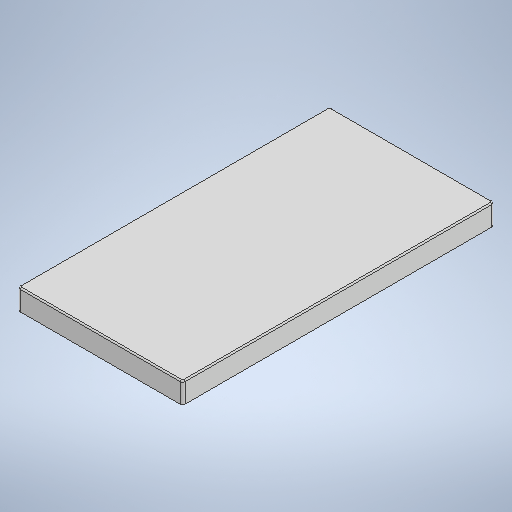
# Autodesk Inventor part: BMS
Saved by Autodesk Inventor 2025.2 (Build 292293000, 293)
## iProperties
Created: 2025-03-19
Part Number: BMS
Material: Generic
Document SubType Name: Modeling
Designer: Tobias
Density: 1 g/cm^3
Appearance: Default
Author: Tobias
Autodesk Inventor part; units mm, degrees
ref_plane "YZ Plane" through (0, 0, 0) normal (1, 0, 0) x (0, 1, 0)
ref_plane "XZ Plane" through (0, 0, 0) normal (0, 1, 0) x (-1, 0, 0)
ref_plane "XY Plane" through (0, 0, 0) normal (0, 0, 1) x (1, 0, 0)
sketch "Sketch1" plane through (0, 0, 0) normal (0, 1, 0) x (-1, 0, 0)
  line L0 (0, 0) -> (63.5, 0)
  line L1 (63.5, 0) -> (63.5, -120)
  line L2 (63.5, -120) -> (0, -120)
  line L3 (0, -120) -> (0, 0)
  dimension "d0" = 63.5
  dimension "d1" = 120
  constraints: 8 end point, 2 parallel, 1 horizontal, 1 perpendicular
  measures "d0" distance of L1.end L2.end
  measures "d1" distance of L0.end L1.end
extrude "Extrusion1" add sketch "Sketch1" along normal blind 8
fillet "Fillet1" radius 1 4 edges at (0, 4, 0) (-63.5, 4, 0) (-63.5, 4, -120) (0, 4, -120)
fillet "Fillet2" radius 0.5 8 edges at (-0.2929, 8, -0.2929) (0, 8, -60) (-0.2929, 8, -119.7071) (-31.75, 8, -120) (-63.2071, 8, -119.7071) (-63.5, 8, -60) (-63.2071, 8, -0.2929) (-31.75, 8, 0)
body "Solid1"
